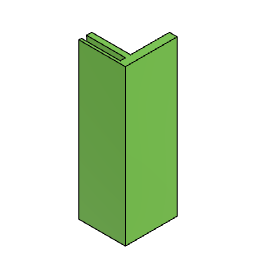
Karton-Beschriftung (Autodesk Fusion 360 design; units mm, degrees)
Autodesk Fusion 360 part; units mm, degrees
sketch "Sketch1" plane through (0, 0, 0) normal (1, 0, 0) x (0, 1, 0)
  line L0 (0, 0) -> (20, 0)
  line L1 (20, 0) -> (20, 60)
  line L2 (20, 60) -> (0, 60)
  line L3 (0, 60) -> (0, 0)
  line L4 (5, 60) -> (5, 0)
  arc A0 (1, 0) -> (1, 60) centre (-448.5, 30) ccw
  arc A1 (3, 0) -> (3, 60) centre (-446.5, 30) ccw
  line L5 (0, 30) -> (5, 30) construction
  line L6 (2, 30) -> (2.3932, 29.5453) construction
  line L7 (4, 30) -> (3.7548, 30.2991) construction
  dimension "d3" = 60
  dimension "d4" = 20
  dimension "d5" = 5
  dimension "d6" = 1
  dimension "d7" = 2
  dimension "d8" = 1
  dimension "d9" = 2
  dimension "d16" = 2
  dimension "d17" = 2
  constraint horizontal L0
  constraint vertical L1
  constraint horizontal L2
  constraint vertical L3
  constraint coincident L0.start L3.end
  constraint coincident L2 L4.start
  constraint coincident L0 L4.end
  constraint perpendicular L0 L4
  constraint coincident L0 A0.start
  constraint coincident L0 A1.start
  constraint coincident L2 A1.end
  constraint coincident L2 A0.end
  constraint midpoint L3 L5.start
  constraint midpoint L4 L5.end
  constraint midpoint A0 L6.start
  constraint midpoint A1 L7.start
  measures "d3" distance of L0.end L1.end
  measures "d4" distance of L0.start L0.end
  measures "d5" distance of L3 L4
  measures "d6" distance of L2.end A0.end
  measures "d7" distance of L4.start A1.end
  measures "d8" distance of L0.start A0.start
  measures "d9" distance of L4.end A1.start
  measures "d16" distance of L5.start L6.start
  measures "d17" distance of L6.start L7.start
extrude "Extrude2" add sketch "Sketch1" along normal blind 3
extrude "Extrude3" add sketch "Sketch1" against normal blind 15 contours L0 L2 L3 A0 | L0 L2 L4 A1
equation "d8 = d6"
equation "d9 = d7"
